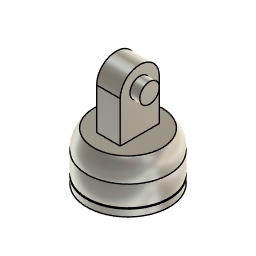
ITEM 2 v1 (Autodesk Fusion 360 design; units mm, degrees)
Autodesk Fusion 360 part; units mm, degrees
note: some values were not read from the file. Set by a fixed rule: which sketch regions a step uses.
sketch "Sketch1" plane through (0, 0, 0) normal (0, 1, 0) x (1, 0, 0)
  line L0 (0, 0) -> (-35, 0)
  line L1 (0, 0) -> (0, 20)
  line L2 (0, 20) -> (-42, 20)
  arc A0 (-42, 20) -> (-35, 0) centre (-17.1273, 17.4804) ccw
  dimension "d1" = 35
  dimension "d2" = 20
  dimension "d3" = 42
  dimension "d4" = 25
  constraint coincident L0.start L1.start
  constraint horizontal L0
  constraint vertical L1
  constraint perpendicular L1 L2
  measures "d1" distance of L0.start L0.end
  measures "d2" distance of L0.start L1.end
  measures "d3" distance of L1.end L2.end
  measures "d4" radius of A0
revolve "Revolve1" add sketch "Sketch1" angle 360 about axis through (0, 0, 0) along (0, 0, -1) in component "Component"
sketch "Sketch2" plane through (0, 0, -20) normal (0, 0, -1) x (1, 0, 0)
  circle A0 centre (0, 0) radius 42
  circle A1 centre (0, 0) radius 39.5
  dimension "d6" = 79
  constraint coincident A0.centre A1.centre
  measures "d6" diameter of A1
extrude "Extrude1" add sketch "Sketch2" along normal blind 1 contours A1 in component "Component"
sketch "Sketch3" plane through (0, 0, 0) normal (1, 0, 0) x (0, 1, 0)
  line L0 (0, -21) -> (0, -41)
  line L1 (0, -41) -> (-42, -41)
  line L2 (0, -21) -> (-40, -21)
  arc A0 (-40, -21) -> (-42, -41) centre (-5.5677, -34.5432) ccw
  dimension "d9" = 20
  dimension "d10" = 42
  dimension "d11" = 40
  dimension "d12" = 37
  constraint vertical L0
  constraint perpendicular L0 L1
  constraint perpendicular L0 L2
  measures "d9" distance of L0.start L0.end
  measures "d10" distance of L0.end L1.end
  measures "d11" distance of L0.start L2.end
  measures "d12" radius of A0
revolve "Revolve2" add sketch "Sketch3" angle 360 about axis through (0, 0, -21) along (0, 0, -1) in component "Component"
sketch "Sketch4" plane through (0, 0, -41) normal (0, 0, -1) x (1, 0, 0)
  circle A0 centre (0, 0) radius 42
  circle A1 centre (0, 0) radius 41
  dimension "d14" = 82
  constraint coincident A0.centre A1.centre
  measures "d14" diameter of A1
extrude "Extrude2" add sketch "Sketch4" along normal blind 1 contours A1 in component "Component"
sketch "Sketch5" plane through (0, 0, -42) normal (0, 0, -1) x (1, 0, 0)
  circle A0 centre (0, 0) radius 41
  circle A1 centre (0, 0) radius 42
  dimension "d17" = 84
  constraint coincident A0.centre A1.centre
  measures "d17" diameter of A1
extrude "Extrude3" add sketch "Sketch5" along normal blind 7 contours A0 | A1 in component "Component"
sketch "Sketch6" plane through (0, 0, -49) normal (0, 0, -1) x (1, 0, 0)
  circle A0 centre (0, 0) radius 42
  circle A1 centre (0, 0) radius 35
  dimension "d20" = 70
  constraint coincident A0.centre A1.centre
  measures "d20" diameter of A1
extrude "Extrude4" add sketch "Sketch6" along normal blind 3 contours A1 in component "Component"
sketch "Sketch7" plane through (0, 0, -49) normal (0, 0, -1) x (1, 0, 0)
  circle A0 centre (0, 0) radius 35
  circle A1 centre (0, 0) radius 42
  line L0 (35, 0.0167) -> (42, 0.0167)
  circle A2 centre (38.5, 0.0167) radius 2.25
  circle A3 centre (38.5, 0.0167) radius 1.5
  dimension "d23" = 4.5
  dimension "d24" = 3
  constraint coincident A0 L0.start
  constraint horizontal L0
  constraint midpoint L0 A2.centre
  constraint concentric A2 A3
  measures "d23" diameter of A2
  measures "d24" diameter of A3
extrude "Extrude5" add sketch "Sketch7" along normal blind 1 contours L0 A2 A3 | L0 A2 A3 in component "Component"
pattern_circular "C-Pattern1" count 16 over 360 about axis through (0, 0, -49) along (0, 0, 1) of "Extrude5" in component "Component"
sketch "Sketch8" plane through (0, 0, 0) normal (0, 0, 1) x (-1, 0, 0)
  circle A0 centre (0, 0) radius 35
  line L0 (12, 20) -> (-12, 20)
  line L1 (-12, 20) -> (-12, -20)
  line L2 (-12, -20) -> (12, -20)
  line L3 (12, -20) -> (12, 20)
  line L4 (12, 20) -> (-12, -20) construction
  line L5 (-12, 20) -> (12, -20) construction
  dimension "d29" = 24
  dimension "d30" = 40
  constraint horizontal L0
  constraint perpendicular L0 L1
  constraint parallel L0 L2
  constraint parallel L1 L3
  constraint coincident L4 A0.centre
  constraint coincident L5 A0.centre
  constraint coincident A0.centre origin
  measures "d29" distance of L1.end L2.end
  measures "d30" distance of L0.end L1.end
extrude "Extrude6" add sketch "Sketch8" along normal blind 42 contours L0 L1 L2 L3 in component "Component"
sketch "Sketch9" plane through (12, 0, 0) normal (1, 0, 0) x (0, 1, 0)
  line L0 (-20, 0) -> (20, 0)
  line L1 (20, 0) -> (20, 42)
  line L2 (20, 42) -> (-20, 42)
  line L3 (-20, 42) -> (-20, 0)
  circle A0 centre (0, 42) radius 20
  constraint midpoint L2 A0.centre
  constraint coincident L2.end A0
extrude "Extrude7" add sketch "Sketch9" against normal blind 24 contours L2 A0 picked at (4.1566, 47.2122) in component "Component"
sketch "Sketch10" plane through (12, 0, 0) normal (1, 0, 0) x (0, 1, 0)
  line L0 (-20, 0) -> (20, 0)
  line L1 (20, 0) -> (20, 42)
  arc A0 (20, 42) -> (-20, 42) centre (0, 42) ccw
  line L2 (-20, 42) -> (-20, 0)
  circle A1 centre (0, 42) radius 10
  dimension "d35" = 20
  constraint concentric A0 A1
  measures "d35" diameter of A1
extrude "Extrude8" add sketch "Sketch10" along normal blind 10 contours A1 in component "Component"
sketch "Sketch11" plane through (0, 0, -52) normal (0, 0, -1) x (1, 0, 0)
  circle A0 centre (0, 0) radius 35
  circle A1 centre (0, 0) radius 10
  dimension "d38" = 20
  constraint coincident A0.centre A1.centre
  measures "d38" diameter of A1
extrude "Extrude9" add sketch "Sketch11" along normal blind 10 contours A1 in component "Component"
component "Component" placed x (1, 0, 0) y (0, 1, 0) z (0, 0, 1) at (0, 0, 0)
